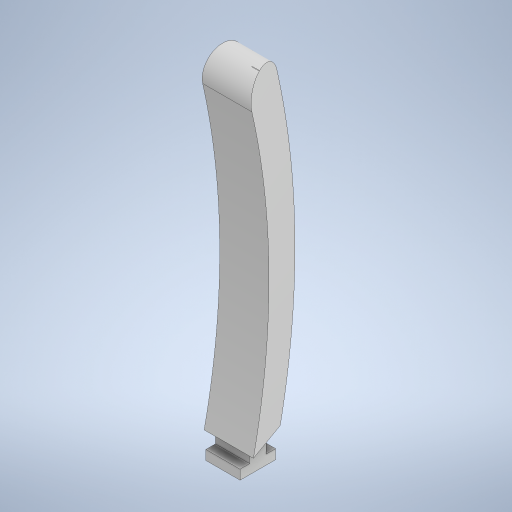
# Autodesk Inventor part: blade_arm
Saved by Autodesk Inventor 2023 (Build 270158000, 158)
## iProperties
Created: 2025-12-21
Part Number: blade_arm
Material: Generic
Document SubType Name: Modeling
Designer: Justin Pascual
Density: 1 g/cm^3
Appearance: Default
Author: Justin Pascual
Autodesk Inventor part; units mm, degrees
ref_plane "YZ Plane" through (0, 0, 0) normal (1, 0, 0) x (0, 1, 0)
ref_plane "XZ Plane" through (0, 0, 0) normal (0, 1, 0) x (-1, 0, 0)
ref_plane "XY Plane" through (0, 0, 0) normal (0, 0, 1) x (1, 0, 0)
sketch "Sketch1" plane through (0, 0, 0) normal (1, 0, 0) x (0, 1, 0)
  arc A0 (0, 0) -> (2.54, -0.5582) centre (57.15, 254) ccw construction
  arc A1 (117.6454, -14.8683) -> (114.3, 0) centre (115.9727, -7.4341) ccw
  line L0 (0, 0) -> (0, -15.5992) construction
  arc A2 (0, -15.5992) -> (2.54, -16.1251) centre (57.15, 254) ccw construction
  line L1 (0, -7.7996) -> (0, -10.8476) construction
  line L2 (2.54, -10.8476) -> (-4.064, -10.8476)
  line L3 (-4.064, -10.8476) -> (-4.064, -14.4036)
  line L4 (-4.064, -14.4036) -> (-7.62, -14.4036)
  line L5 (-7.62, -14.4036) -> (-7.62, -7.7996)
  line L6 (2.54, -7.7996) -> (-7.62, -7.7996) construction
  line L7 (0, -7.7996) -> (0, -4.7516) construction
  line L8 (2.54, -4.7516) -> (-4.064, -4.7516)
  line L9 (-4.064, -4.7516) -> (-4.064, -1.1956)
  line L10 (-4.064, -1.1956) -> (-7.62, -1.1956)
  line L11 (-7.62, -1.1956) -> (-7.62, -7.7996)
  line L12 (0, -7.7996) -> (2.54, -7.7996) construction
  line L13 (2.54, -0.5582) -> (2.54, -4.7516)
  line L14 (2.54, -10.8476) -> (2.54, -16.1251)
  arc A3 (2.54, -16.1251) -> (117.6454, -14.8683) centre (57.15, 254) ccw
  arc A4 (2.54, -0.5582) -> (114.3, 0) centre (57.15, 254) ccw
  point P0 (57.15, -6.35)
  point P1 (0, -10.8476)
  point P2 (0, -4.7516)
  dimension "d0" = 57.15
  dimension "d1" = 114.3
  dimension "d3" = 6.35
  dimension "d8" = 3.048
  dimension "d9" = 6.604
  dimension "d10" = 3.556
  dimension "d11" = 3.556
  dimension "d56" = 2.54
  constraints: 30 end point, 12 point on circle, 5 centre point, 4 symmetric about line, 3 perpendicular, 2 vertical, 1 coincident, 1 horizontal, 1 tangent
  measures "d0" horizontal distance of point (57.15, -6.35) A1.end
  measures "d1" distance of A1.end L0.start
  measures "d3" vertical distance of A1.end point (57.15, -6.35)
  measures "d8" distance of L1.start L1.end
  measures "d9" distance of L2.start L2.end
  measures "d10" distance of L2.end L3.end
  measures "d11" distance of L3.end L4.end
  measures "d56" distance of L12.start L12.end
extrude "Extrusion2" add sketch "Sketch1" along normal blind 12.7
sketch "Sketch5" plane through (0, 0, 0) normal (-1, 0, 0) x (0, 0, 1)
  arc A0 (0, 114.3) -> (-14.8683, 117.6454) centre (-7.4341, 115.9727) ccw projected
  arc A1 (-7.4341, 115.9727) -> (-8.4072, 2.8323) centre (254, 57.15) ccw
  arc A2 (0, 114.3) -> (-0.5582, 2.54) centre (254, 57.15) ccw projected
  arc A3 (-5.6559, 123.3823) -> (-7.4341, 115.9727) centre (254, 57.15) ccw
  point P0 (0, 0)
  constraints: 6 point on circle, 2 centre point, 1 concentric
ref_plane "Work Plane3" through (0, 123.3823, -5.6559) normal (0, 0.9723901, 0.2333612) x (-1, 0, 0)
sketch "Sketch7" plane through (12.7, 0, 0) normal (1, 0, 0) x (0, 0, -1)
  arc A0 (14.8683, 117.6454) -> (0, 114.3) centre (7.4341, 115.9727) ccw projected
  point P0 (0, 0)
sketch "Sketch8" plane through (0, 0, 0) normal (-1, 0, 0) x (0, 0, 1)
  arc A0 (0, 114.3) -> (-14.8683, 117.6454) centre (-7.4341, 115.9727) ccw projected
  point P0 (0, 0)
ref_plane "Work Plane4" through (0, 114.3, 0) normal (0, 0.9756098, 0.2195122) x (1, 0, 0)
sketch "Sketch9" plane through (0, 114.3, 0) normal (0, 0.9756098, 0.2195122) x (1, 0, 0)
  line L0 (0, 0) -> (12.7, 0) projected
  line L1 (0, 0) -> (-5.588, 0)
  line L2 (0, -8.8008) -> (0, 15.24) projected
  line L3 (0, 15.24) -> (0, 15.24)
  line L4 (0, 15.24) -> (-5.588, 0)
  point P0 (0, -25.0902)
  dimension "d65" = 5.588
  dimension "d66" = 0
  constraints: 6 end point, 2 horizontal
  measures "d65" distance of L0.start L1.end
  measures "d66" distance of L2.end L3.end
sketch "Sketch10" plane through (0, 0, 0) normal (-1, 0, 0) x (0, 0, 1)
  arc A0 (0, 114.3) -> (-14.8683, 117.6454) centre (-7.4341, 115.9727) ccw projected
  arc A1 (-7.4341, 115.9727) -> (-7.8923, 0.4017) centre (254, 57.15) ccw
  arc A2 (0, 114.3) -> (-0.5582, 2.54) centre (254, 57.15) ccw projected
  arc A3 (-5.6559, 123.3823) -> (-7.4341, 115.9727) centre (254, 57.15) ccw
  line L0 (-10.8476, 2.54) -> (-16.1251, 2.54) projected
  line L1 (-0.5582, 2.54) -> (-4.7516, 2.54) projected
  line L2 (-10.8476, -4.064) -> (-10.8476, 2.54) projected
  line L3 (-10.8476, 0.4017) -> (-4.7598, 0.4017)
  point P0 (0, 0)
  constraints: 6 point on circle, 2 centre point, 2 concentric, 2 end point, 2 point on line, 1 horizontal
sweep "Sweep4" add profiles "Sketch9" path "Sketch10" path curves A3 A1
ref_plane "Work Plane5" through (-12.7, 0, 0) normal (1, 0, 0) x (0, 0, -1)
sketch "Sketch11" plane through (-12.7, 0, 0) normal (1, 0, 0) x (0, 0, -1)
  arc A0 (0.5582, 2.54) -> (0, 114.3) centre (-254, 57.15) ccw projected
  arc A1 (16.1251, 2.54) -> (14.8683, 117.6454) centre (-254, 57.15) ccw projected
  arc A2 (16.1251, 2.54) -> (14.8683, 117.6454) centre (-254, 57.15) ccw projected
  arc A3 (14.8683, 117.6454) -> (0, 114.3) centre (7.4341, 115.9727) ccw projected
  arc A4 (0.5582, 2.54) -> (0, 114.3) centre (-254, 57.15) ccw projected
  line L0 (0.5582, 2.54) -> (4.7516, 2.54) projected
  line L1 (4.7516, 2.54) -> (4.7516, -4.064) projected
  line L2 (4.7516, -4.064) -> (1.1956, -4.064) projected
  line L3 (1.1956, -4.064) -> (1.1956, -7.62) projected
  line L4 (1.1956, -7.62) -> (14.4036, -7.62) projected
  line L5 (14.4036, -7.62) -> (14.4036, -4.064) projected
  line L6 (14.4036, -4.064) -> (10.8476, -4.064) projected
  line L7 (10.8476, -4.064) -> (10.8476, 2.54) projected
  line L8 (10.8476, 2.54) -> (16.1251, 2.54) projected
  line L9 (-43.4554, -29.2005) -> (78.0599, -29.2005)
  line L10 (78.0599, -29.2005) -> (78.0599, 145.7037)
  line L11 (78.0599, 145.7037) -> (-43.4554, 145.7037)
  line L12 (-43.4554, 145.7037) -> (-43.4554, -29.2005)
  point P0 (0, 0)
  point P1 (0, 114.3)
  point P2 (14.8683, 117.6454)
  point P3 (16.1251, 2.54)
  constraints: 8 end point, 2 parallel, 1 horizontal, 1 perpendicular
extrude "Extrusion3" cut sketch "Sketch11" along normal blind 12.7
sketch "Sketch12" plane through (0, 0, 0) normal (-1, 0, 0) x (0, 0, 1)
  arc A0 (-14.8683, 117.6454) -> (-16.1251, 2.54) centre (254, 57.15) ccw construction
  arc A1 (0, 114.3) -> (-14.8683, 117.6454) centre (-7.4341, 115.9727) ccw projected
  arc A2 (0, 114.3) -> (-0.5582, 2.54) centre (254, 57.15) ccw construction
  line L0 (-0.5582, 2.54) -> (-4.7516, 2.54) construction
  line L1 (-4.7516, 2.54) -> (-4.7516, -4.064) projected
  line L2 (-4.7516, -4.064) -> (-1.1956, -4.064) projected
  line L3 (-1.1956, -4.064) -> (-1.1956, -7.62) projected
  line L4 (-1.1956, -7.62) -> (-14.4036, -7.62) projected
  line L5 (-14.4036, -7.62) -> (-14.4036, -4.064) projected
  line L6 (-14.4036, -4.064) -> (-10.8476, -4.064) projected
  line L7 (-10.8476, -4.064) -> (-10.8476, 2.54) projected
  line L8 (-10.8476, 2.54) -> (-16.1251, 2.54) construction
  line L9 (-16.1251, 2.54) -> (-16.1251, 2.54)
  line L10 (-4.7516, 2.54) -> (-10.8476, 2.54)
  point P0 (0, 0)
  constraints: 4 end point, 1 collinear, 1 horizontal
extrude "Extrusion4" cut sketch "Sketch12" along normal blind 12.7
fillet "Fillet1" [suppressed]
ref_plane "Work Plane6" through (6.35, 0, 0) normal (1, 0, 0) x (0, 0, -1)
mirror "Mirror1" about plane through (6.35, 0, 0) normal (1, 0, 0) remove original yes
fillet "Fillet4" [suppressed]
equation "\"d0\" = 0.5 * d1"
body "Solid2"
